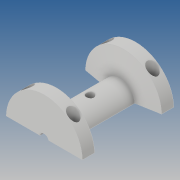
# Autodesk Inventor part: demi_tambour
Saved by Autodesk Inventor 2019 (Build 230136000, 136)
## iProperties
Created: 2020-07-07
Part Number: demi_tambour
Material: Générique
Document SubType Name: Modeling
Designer: Theo
Density: 1 g/cm^3
Appearance: Par défaut
Author: Theo
Autodesk Inventor part; units mm, degrees
ref_plane "YZ Plane" through (0, 0, 0) normal (1, 0, 0) x (0, 1, 0)
ref_plane "XZ Plane" through (0, 0, 0) normal (0, 1, 0) x (-1, 0, 0)
sketch "Esquisse1" plane through (0, 0, 0) normal (1, 0, 0) x (0, 1, 0)
  line L0 (0, 0) -> (0, -46.4485)
  line L1 (2.875, 0) -> (25, 0)
  line L2 (25, 0) -> (25, -8)
  line L3 (2.875, 0) -> (2.875, -60)
  line L4 (25, -8) -> (10, -10.6449)
  line L5 (10, -10.6449) -> (10, -49.3551)
  line L6 (10, -49.3551) -> (25, -52)
  line L7 (25, -52) -> (25, -60)
  line L8 (2.875, -60) -> (25, -60)
  dimension "d0" = 5.75
  dimension "d1" = 50
  dimension "d2" = 20
  dimension "d3" = 100
  dimension "d4" = 8
  dimension "d5" = 100
  dimension "d6" = 60
  dimension "d7" = 15
  dimension "d8" = 38.7102
  constraints: 18 end point, 5 vertical, 2 collinear, 2 horizontal, 1 point on line
  measures "d0" diameter of L3 L0
  measures "d1" diameter of L2 L0
  measures "d2" diameter of L5 L0
  measures "d3" angle of L5 L4
  measures "d4" distance of L1.end L2.end
  measures "d5" angle of L5 L6
  measures "d6" distance between parallel lines of L1 L8
  measures "d7" distance between parallel lines of L2 L5
  measures "d8" distance of L4.end L5.end
revolve "Révolution1" add sketch "Esquisse1" angle 360 about axis through (0, 0, 0) along (0, 0, -1)
sketch "Esquisse2" plane through (0, 0, 0) normal (0, 0, 1) x (1, 0, 0)
  circle A0 centre (0, 0) radius 25 projected
  line L0 (-25, 0.5) -> (25, 0.5)
  line L1 (25, 0.5) -> (25, -25)
  line L2 (25, -25) -> (-25, -25)
  line L3 (-25, -25) -> (-25, 0.5)
  point P0 (-25, 0)
  point P1 (25, 0)
  dimension "d42" = 0.5
  constraints: 8 end point, 3 tangent, 2 parallel, 2 point on circle, 1 horizontal, 1 perpendicular
  measures "d42" distance from line of L0 A0.centre
extrude "Extrusion1" cut sketch "Esquisse2" against normal up to surface (60 mm away) contours A0 L0 | L1 L2 A0 | A0 L0 L1 | L2 L3 A0 | A0 L3 L0 picked at (-6.5153, -4.8624)
sketch "Esquisse3" plane through (-25, 0.5, 0) normal (0, -1, 0) x (1, 0, 0)
  line L0 (0, -52) -> (15, -49.3551) projected
  line L1 (0, -60) -> (0, -52) projected
  line L2 (22.125, -60) -> (0, -60) projected
  line L3 (22.125, 0) -> (22.125, -60) projected
  line L4 (0, 0) -> (22.125, 0) projected
  line L5 (0, -8) -> (0, 0) projected
  line L6 (15, -10.6449) -> (0, -8) projected
  line L7 (15, -49.3551) -> (15, -10.6449) projected
  line L8 (35, -49.3551) -> (50, -52) projected
  line L9 (35, -10.6449) -> (35, -49.3551) projected
  line L10 (50, -8) -> (35, -10.6449) projected
  line L11 (50, 0) -> (50, -8) projected
  line L12 (27.875, 0) -> (50, 0) projected
  line L13 (27.875, -60) -> (27.875, 0) projected
  line L14 (50, -60) -> (27.875, -60) projected
  line L15 (50, -52) -> (50, -60) projected
  line L16 (22.1688, -60) -> (27.8312, -60) projected
  line L17 (22.1688, 0) -> (27.8312, 0) projected
  circle A0 centre (25, -30) radius 2.5
  line L18 (27.8312, -60) -> (27.8312, 0) projected
  line L19 (22.1688, 0) -> (22.1688, -60) projected
  point P0 (25, 0)
  point P1 (22.125, 0)
  point P2 (27.875, 0)
  point P3 (25, 0)
  dimension "d13" = 60
  dimension "d14" = 30
  dimension "d15" = 5
  constraints: 1 centre point, 1 midpoint, 1 vertical alignment
  measures "d13" distance between parallel lines of L14 L12
  measures "d14" distance from line of L14 A0.centre
  measures "d15" diameter of A0
extrude "Extrusion2" cut sketch "Esquisse3" against normal up to surface contours A0
ref_plane "Plan de construction2" through (0, 25, -60) normal (0, 1, 0) x (-1, 0, 0)
sketch "Esquisse6" plane through (0, 25, -60) normal (0, 1, 0) x (-1, 0, 0)
  line L0 (24.995, 0) -> (-24.995, 0) projected
  line L1 (24.995, 8) -> (-24.995, 8) projected
  line L2 (24.995, 52) -> (-24.995, 52) projected
  line L3 (24.995, 60) -> (-24.995, 60) projected
  line L4 (-24.995, 60) -> (-24.995, 52) projected
  line L5 (24.995, 52) -> (24.995, 60) projected
  line L6 (-24.995, 8) -> (-24.995, 0) projected
  line L7 (24.995, 0) -> (24.995, 8) projected
  point P0 (0, 60)
  point P1 (25, 8)
  point P2 (25, 0)
  point P3 (-25, 0)
  point P4 (-25, 8)
  point P5 (25, 60)
  point P6 (25, 52)
  point P7 (-25, 52)
  point P8 (-25, 60)
  point P9 (-15, 4)
  point P10 (15, 4)
  point P11 (15, 56)
  point P12 (-15, 56)
  dimension "d31" = 8
  dimension "d32" = 4
  dimension "d33" = 4
  constraints: 2 horizontal alignment, 2 vertical alignment
  measures "d31" distance of point (25, 60) point (25, 52)
  measures "d32" distance from line of L3 point (-15, 56)
  measures "d33" distance from line of L0 point (-15, 4)
hole "Perçage2" at (15, 25, -56) at (-15, 25, -56) at (-15, 25, -4) at (15, 25, -4) direction (0, -1, 0) diameter 4 end through all counterbore diameter 6.9 counterbore depth 21
equation "\"d5\" = d3"
equation "\"d14\" = 0.5 * d13"
equation "\"d32\" = 0.5 * d31"
equation "\"d33\" = d32"
